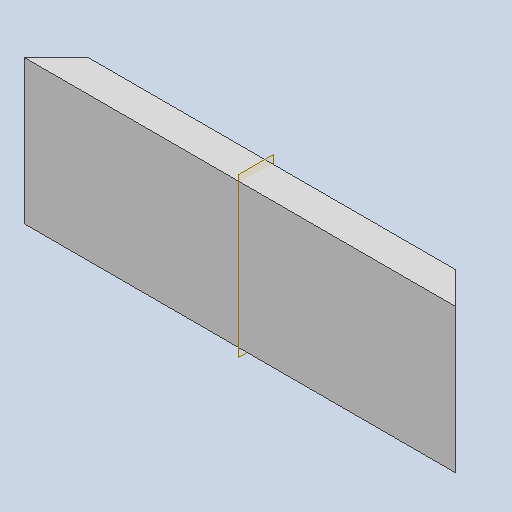
# Autodesk Inventor part: PDMS Chamber-Mold-V8-Left_Right-Wall Steven
Saved by Autodesk Inventor 2022 (Build 260153000, 153)
## iProperties
Created: 2021-11-29
Part Number: PDMS Chamber-Mold-V8-Left_Right-Wall Steven
Material: Generic
Document SubType Name: Modeling
Designer: Hirota Lab
Density: 1 g/cm^3
Appearance: Default
Author: Hirota Lab
Autodesk Inventor part; units mm, degrees
ref_plane "XZ Plane" through (0, 0, 0) normal (0, 1, 0) x (-1, 0, 0)
ref_plane "XY Plane" through (0, 0, 0) normal (0, 0, 1) x (1, 0, 0)
sketch "Sketch1" plane through (0, 0, 0) normal (0, 1, 0) x (-1, 0, 0)
  line L0 (0, 0) -> (54, 0)
  line L1 (4, -4) -> (50, -4)
  line L2 (0, -4) -> (50, -4) construction
  line L3 (50, -4) -> (54, 0)
  line L4 (0, 0) -> (4, -4)
  dimension "d0" = 54
  dimension "d1" = 4
  dimension "d3" = 0
  constraints: 10 end point, 3 horizontal, 1 perpendicular
  measures "d0" distance of L0.start L0.end
  measures "d1" distance of L0.start L2.start
  measures "d3" distance between parallel lines of L1 L2
extrude "Extrusion1" add sketch "Sketch1" along normal blind 17
sketch "Sketch2" plane through (-4, 0, -4) normal (0, 0, -1) x (-1, 0, 0)
  line L0 (-4, 0) -> (-4, 17) projected
  line L1 (50, 0) -> (50, 17) projected
  line L2 (-4, 2) -> (50, 2)
  line L3 (50, 2) -> (50, 6.1)
  line L4 (50, 6.1) -> (-4, 6.1)
  line L5 (-4, 6.1) -> (-4, 2)
  line L6 (0, 0) -> (46, 0) projected
  point P0 (-4, 6.1)
  dimension "d6" = 4.1
  dimension "d7" = 2
  constraints: 8 end point, 2 parallel, 2 point on line, 1 horizontal, 1 perpendicular
  measures "d6" distance of L3.end L2.end
  measures "d7" distance between parallel lines of L6 L2
sketch "Sketch3" plane through (0, 17, 0) normal (0, 1, 0) x (1, 0, 0)
  line L0 (-50, 4) -> (-54, 0) projected
  line L1 (-54, 0) -> (0, 0) projected
  line L2 (0, 0) -> (-4, 4) projected
  line L3 (-4, 4) -> (-50, 4) projected
extrude "Extrusion2" add sketch "Sketch3" along normal blind 1.05
extrude "Extrusion3" cut sketch "Sketch2" against normal blind 2.05
ref_plane "Work Plane1" through (-27, 0, 0) normal (1, 0, 0) x (0, 1, 0)
body "Solid1"
